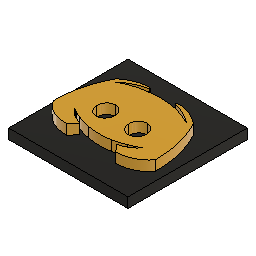
icon_discord (Autodesk Fusion 360 design; units mm, degrees)
Autodesk Fusion 360 part; units mm, degrees
sketch "Sketch1" plane through (0, 0, 0) normal (0, 0, 1) x (1, 0, 0)
  line L0 (5.95, -5.95) -> (-5.95, -5.95)
  line L1 (-5.95, -5.95) -> (-5.95, 5.95)
  line L2 (-5.95, 5.95) -> (5.95, 5.95)
  line L3 (5.95, 5.95) -> (5.95, -5.95)
  line L4 (5.95, -5.95) -> (-5.95, 5.95) construction
  line L5 (-5.95, -5.95) -> (5.95, 5.95) construction
  spline S0 degree 3 poles (1.569, 0.3676) (1.0713, 0.3676) (0.6784, -0.0602) (0.6784, -0.5928) knots 0 0 0 0 1 1 1 1
  spline S1 degree 3 poles (0.6784, -0.5928) (0.6784, -1.1254) (1.08, -1.5532) (1.569, -1.5532) knots 0 0 0 0 1 1 1 1
  spline S2 degree 3 poles (1.569, -1.5532) (2.0667, -1.5532) (2.4596, -1.1254) (2.4596, -0.5928) knots 0 0 0 0 1 1 1 1
  spline S3 degree 3 poles (2.4596, -0.5928) (2.4596, -0.0602) (2.0579, 0.3676) (1.569, 0.3676) knots 0 0 0 0 1 1 1 1
  spline S4 degree 3 poles (-1.6179, 0.3676) (-2.1156, 0.3676) (-2.5085, -0.0602) (-2.5085, -0.5928) knots 0 0 0 0 1 1 1 1
  spline S5 degree 3 poles (-2.5085, -0.5928) (-2.5085, -1.1254) (-2.1069, -1.5532) (-1.6179, -1.5532) knots 0 0 0 0 1 1 1 1
  spline S6 degree 3 poles (-1.6179, -1.5532) (-1.1202, -1.5532) (-0.7273, -1.1254) (-0.7273, -0.5928) knots 0 0 0 0 1 1 1 1
  spline S7 degree 3 poles (-0.7273, -0.5928) (-0.7186, -0.0602) (-1.1202, 0.3676) (-1.6179, 0.3676) knots 0 0 0 0 1 1 1 1
  spline S8 degree 2 poles (2.4421, -3.6749) (2.1278, -3.2995) (1.8659, -2.9764) knots 0 0 0 1 1 1
  spline S9 degree 2 poles (1.8659, -2.9764) (3.0096, -2.6534) (3.4462, -1.9461) knots 0 0 0 1 1 1
  spline S10 degree 3 poles (3.4462, -1.9461) (3.0882, -2.1819) (2.7477, -2.3478) (2.4421, -2.4613) knots 0 0 0 0 1 1 1 1
  spline S11 degree 3 poles (2.4421, -2.4613) (2.0056, -2.6446) (1.5865, -2.7581) (1.1761, -2.8367) knots 0 0 0 0 1 1 1 1
  spline S12 degree 3 poles (1.1761, -2.8367) (0.3379, -2.9939) (-0.4305, -2.9502) (-1.0853, -2.828) knots 0 0 0 0 1 1 1 1
  spline S13 degree 3 poles (-1.0853, -2.828) (-1.583, -2.7319) (-2.0108, -2.601) (-2.3688, -2.4525) knots 0 0 0 0 1 1 1 1
  spline S14 degree 3 poles (-2.3688, -2.4525) (-2.5696, -2.374) (-2.7879, -2.2779) (-3.0062, -2.1557) knots 0 0 0 0 1 1 1 1
  spline S15 degree 3 poles (-3.0062, -2.1557) (-3.0324, -2.1382) (-3.0586, -2.1295) (-3.0848, -2.112) knots 0 0 0 0 1 1 1 1
  spline S16 degree 3 poles (-3.0848, -2.112) (-3.1022, -2.1033) (-3.111, -2.0946) (-3.1197, -2.0946) knots 0 0 0 0 1 1 1 1
  spline S17 degree 2 poles (-3.1197, -2.0946) (-3.2769, -2.0073) (-3.3642, -1.9461) knots 0 0 0 1 1 1
  spline S18 degree 2 poles (-3.3642, -1.9461) (-2.9451, -2.6359) (-1.8362, -2.9677) knots 0 0 0 1 1 1
  spline S19 degree 2 poles (-1.8362, -2.9677) (-2.0981, -3.2995) (-2.4212, -3.6837) knots 0 0 0 1 1 1
  spline S20 degree 2 poles (-2.4212, -3.6837) (-4.3508, -3.6225) (-5.0842, -2.3652) knots 0 0 0 1 1 1
  spline S21 degree 2 poles (-5.0842, -2.3652) (-5.0842, 0.42) (-3.8269, 2.6814) knots 0 0 0 1 1 1
  spline S22 degree 2 poles (-3.8269, 2.6814) (-2.5696, 3.6157) (-1.3822, 3.5895) knots 0 0 0 1 1 1
  line L6 (-1.3822, 3.5895) -> (-1.2949, 3.4847)
  spline S23 degree 2 poles (-1.2949, 3.4847) (-2.8665, 3.0394) (-3.5824, 2.3496) knots 0 0 0 1 1 1
  spline S24 degree 2 poles (-3.5824, 2.3496) (-3.3904, 2.4544) (-3.0673, 2.5941) knots 0 0 0 1 1 1
  spline S25 degree 3 poles (-3.0673, 2.5941) (-2.1331, 3.0045) (-1.3909, 3.1093) (-1.0853, 3.1442) knots 0 0 0 0 1 1 1 1
  spline S26 degree 3 poles (-1.0853, 3.1442) (-1.0329, 3.1529) (-0.9893, 3.1616) (-0.9369, 3.1616) knots 0 0 0 0 1 1 1 1
  spline S27 degree 3 poles (-0.9369, 3.1616) (-0.4043, 3.2315) (0.1982, 3.249) (0.8268, 3.1791) knots 0 0 0 0 1 1 1 1
  spline S28 degree 3 poles (0.8268, 3.1791) (1.6563, 3.0831) (2.5469, 2.8386) (3.4549, 2.3496) knots 0 0 0 0 1 1 1 1
  spline S29 degree 2 poles (3.4549, 2.3496) (2.7652, 3.0045) (1.2809, 3.4498) knots 0 0 0 1 1 1
  line L7 (1.2809, 3.4498) -> (1.4031, 3.5895)
  spline S30 degree 2 poles (1.4031, 3.5895) (2.5993, 3.6157) (3.8478, 2.6814) knots 0 0 0 1 1 1
  spline S31 degree 2 poles (3.8478, 2.6814) (5.1051, 0.42) (5.1051, -2.3652) knots 0 0 0 1 1 1
  spline S32 degree 3 poles (5.1051, -2.3652) (5.1051, -2.3565) (4.3717, -3.6138) (2.4421, -3.6749) knots 0 0 0 0 1 1 1 1
  dimension "d1" = 11.9
  dimension "d2" = 11.9
  constraint perpendicular L0 L1
  constraint parallel L1 L3
  constraint coincident L4 origin
  constraint coincident L5 origin
  measures "d1" distance of L1.end L2.end
  measures "d2" distance of L0.end L1.end
extrude "Extrude1" add sketch "Sketch1" against normal blind 1 contours L0 L1 L2 L3 | S0 S1 S2 S3 | S4 S5 S6 S7 | S8 S9 S10 S11 S12 S13 S14 S15 S16 S17 S18 S19 S20 S21 S22 L6 S23 S24 S25 S26 S27 S28 S29 L7 S30 S31 S32
extrude "Extrude3" add sketch "Sketch1" along normal blind 1 contours S8 S9 S10 S11 S12 S13 S14 S15 S16 S17 S18 S19 S20 S21 S22 L6 S23 S24 S25 S26 S27 S28 S29 L7 S30 S31 S32
